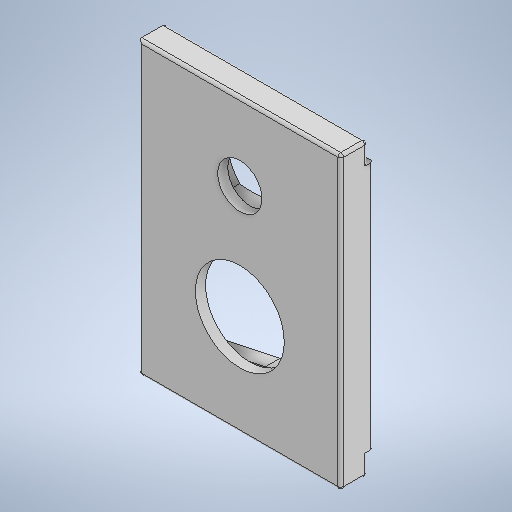
# Autodesk Inventor part: 1mL + 20 mL Luer-Lok 001
Saved by Autodesk Inventor 2025 (Build 290162000, 162)
## iProperties
Created: 2024-04-08
Part Number: 1mL + 20 mL Luer-Lok 001
Material: Generisch
Document SubType Name: Modeling
Designer: noahm
Density: 1 g/cm^3
Appearance: Vorgabe
Author: noahm
Autodesk Inventor part; units mm, degrees
ref_plane "YZ Plane" through (0, 0, 0) normal (1, 0, 0) x (0, 1, 0)
ref_plane "XZ Plane" through (0, 0, 0) normal (0, 1, 0) x (-1, 0, 0)
ref_plane "XY Plane" through (0, 0, 0) normal (0, 0, 1) x (1, 0, 0)
sketch "Skizze1" plane through (0, 0, 0) normal (0, 1, 0) x (-1, 0, 0)
  line L0 (-25, -36) -> (25, -36)
  line L1 (25, -36) -> (25, 36)
  line L2 (25, 36) -> (-25, 36)
  line L3 (-25, 36) -> (-25, -36)
  line L4 (-25, -36) -> (25, 36) construction
  line L5 (25, -36) -> (-25, 36) construction
  circle A0 centre (0, 17) radius 5.5
  circle A1 centre (0, -11) radius 11
  point P0 (0, 0)
  point P1 (0, 36)
  point P2 (0, -36)
  dimension "d0" = 72
  dimension "d1" = 50
  dimension "d2" = 11
  dimension "d3" = 19
  dimension "d4" = 25
  dimension "d5" = 22
  dimension "d6" = 25
  dimension "d7" = 25
  constraints: 12 end point, 4 midpoint, 2 centre point, 2 parallel, 1 horizontal, 1 perpendicular
  measures "d0" distance of L0.end L1.end
  measures "d1" distance of L1.end L2.end
  measures "d2" diameter of A0
  measures "d3" distance of point (0, 36) A0.centre
  measures "d4" distance from line of L1 A0.centre
  measures "d5" diameter of A1
  measures "d6" distance of point (0, -36) A1.centre
  measures "d7" distance from line of L1 A1.centre
extrude "Extrusion1" add sketch "Skizze1" along normal blind 2.5
sketch "Skizze2" plane through (0, 2.5, 0) normal (0, 1, 0) x (1, 0, 0)
  circle A0 centre (0, 11) radius 11
  circle A1 centre (0, -17) radius 5.5
  line L0 (-8.046738, -9.5) -> (0, -10.112591)
  line L1 (0, -10.112591) -> (8.046738, -9.5)
  line L2 (12.459936, -4) -> (0, -3.051436)
  line L3 (0, -3.051436) -> (-12.459936, -4)
  line L4 (-8.046738, -24.5) -> (0, -23.906364)
  line L5 (0, -23.906364) -> (8.046738, -24.5)
  line L6 (-12.459936, 26) -> (0, 25.080787)
  line L7 (0, 25.080787) -> (12.459936, 26)
  arc A2 (8.046738, -24.5) -> (8.046738, -9.5) centre (0, -17) ccw
  arc A3 (-8.046738, -9.5) -> (-8.046738, -24.5) centre (0, -17) ccw
  arc A4 (12.459936, -4) -> (12.459936, 26) centre (0, 11) ccw
  arc A5 (-12.459936, 26) -> (-12.459936, -4) centre (0, 11) ccw
  line L8 (-25, -36) -> (25, -36)
  line L9 (-25, 36) -> (-25, -36)
  line L10 (25, -36) -> (-25, -36)
  line L11 (-25, -36) -> (-25, 36)
  line L12 (-25, 36) -> (25, 36)
  line L13 (25, 36) -> (25, -36)
  point P0 (0, 0)
  point P1 (0, -9.5)
  point P2 (0, -24.5)
  point P3 (0, 26)
  dimension "d12" = 0
  dimension "d13" = 0
  dimension "d14" = 7.5
  dimension "d16" = 7.5
  dimension "d17" = 15
  constraints: 24 end point, 8 point on circle, 6 parallel, 4 centre point, 1 horizontal, 1 perpendicular, 1 vertical alignment
  measures "d12" distance of point (0, 11) A4.centre
  measures "d13" distance of A1.centre A2.centre
  measures "d14" distance of A2.centre point (0, -9.5)
  measures "d16" distance of A2.centre point (0, -24.5)
  measures "d17" distance of A4.centre point (0, 26)
extrude "Extrusion2" add sketch "Skizze2" along normal blind 1.7 contours L9 L12 L13 L8
sketch "Skizze3" plane through (0, 4.2, 0) normal (0, 1, 0) x (1, 0, 0)
  line L0 (-25, -36) -> (25, -36) projected
  line L1 (25, 36) -> (-25, 36) projected
  line L2 (-25, -36) -> (25, -36)
  line L3 (25, -36) -> (25, 36)
  line L4 (25, 36) -> (-25, 36)
  line L5 (-25, 36) -> (-25, -36)
  point P0 (0, 0)
  constraints: 8 end point, 2 parallel, 1 horizontal, 1 perpendicular
extrude "Extrusion3" add sketch "Skizze3" along normal blind 3.8
sketch "Skizze4" plane through (0, 8, 0) normal (0, 1, 0) x (1, 0, 0)
  arc A0 (-8.046738, -9.5) -> (-10.944133, -18.107223) centre (0, -17) ccw
  arc A1 (8.046738, -24.5) -> (10.994414, -16.649483) centre (0, -17) ccw
  arc A2 (0.069499, -10.122825) -> (-0.070045, -10.107258) centre (-0.221864, -12.101488) ccw
  arc A3 (132.908051, -33.706836) -> (133.210878, -29.728206) centre (132.919515, -31.706869) ccw
  arc A4 (12.459811, -3.99999) -> (19.29294, 13.833232) centre (-0.000137, 11) ccw
  line L0 (12.459811, -3.99999) -> (12.459936, -4)
  arc A5 (-4.699403, -1.782332) -> (-4.576398, -1.84238) centre (-3.76103, -0.016134) ccw
  arc A6 (4.726856, 23.857004) -> (4.581609, 23.857004) centre (4.654232, 21.858323) ccw
  arc A7 (0.173536, 25.036036) -> (-0.178728, 25.093972) centre (-0.325875, 23.099393) ccw
  arc A8 (-0.17125, -3.007275) -> (0.176342, -3.064861) centre (0.328161, -1.070632) ccw
  line L1 (19.293045, 13.832979) -> (19.293151, 13.832726) construction
  spline S0 degree 2 poles (19.29294, 13.833232) (19.293045, 13.832979) (19.293151, 13.832726) knots 0 0 0 1 1 1
  line L2 (19.293151, 13.832726) -> (19.293006, 13.832782)
  line L3 (-1.683069, 21.870477) -> (-1.988258, 21.987421)
  arc A9 (12.459936, -4) -> (19.293151, 13.832726) centre (0, 11) ccw
  arc A10 (-12.459936, 26) -> (-19.465197, 9.835475) centre (0, 11) ccw
  line L4 (-2.63509, -24) -> (-2.613775, -24.002826) construction
  spline S1 degree 2 poles (-2.63509, -24) (-2.613775, -24.002826) (-2.592502, -24.005641) knots 0 0 0 1 1 1
  line L5 (2.590414, -10) -> (2.622634, -9.912932)
  line L6 (2.625489, -10.025506) -> (2.590414, -10)
  line L7 (-2.63509, -24) -> (-3.652778, -23.822078) construction
  line L8 (-3.652778, -23.822078) -> (-10.555962, -19.321714) construction
  line L9 (-10.555962, -19.321714) -> (-10.944133, -18.107223) construction
  spline S2 degree 3 poles (-2.63509, -24) (-3.652778, -23.822078) (-10.555962, -19.321714) (-10.944133, -18.107223) knots 1 1 1 1 2 2 2 2
  line L10 (-2.613775, -24.002826) -> (-2.592502, -24.005641) construction
  line L11 (-2.613775, -24.002826) -> (-2.047447, -24.5) construction
  line L12 (-2.047447, -24.5) -> (7.063429, -25.007938) construction
  line L13 (7.063429, -25.007938) -> (8.046738, -24.5) construction
  spline S3 degree 3 poles (-2.613775, -24.002826) (-2.047447, -24.5) (7.063429, -25.007938) (8.046738, -24.5) knots 1 1 1 1 2 2 2 2
  line L14 (-8.046738, -9.5) -> (-7.10437, -8.961841) construction
  line L15 (-7.10437, -8.961841) -> (1.902827, -9.5) construction
  line L16 (1.902827, -9.5) -> (2.590414, -10) construction
  spline S4 degree 3 poles (-8.046738, -9.5) (-7.10437, -8.961841) (1.902827, -9.5) (2.590414, -10) knots 1 1 1 1 2 2 2 2
  line L17 (2.625489, -10.025506) -> (3.48361, -9.847387) construction
  line L18 (3.48361, -9.847387) -> (10.59265, -15.534689) construction
  line L19 (10.59265, -15.534689) -> (10.994414, -16.649483) construction
  spline S5 degree 3 poles (2.625489, -10.025506) (3.48361, -9.847387) (10.59265, -15.534689) (10.994414, -16.649483) knots 1 1 1 1 2 2 2 2
  line L20 (19.29294, 13.833232) -> (19.293045, 13.832979) construction
  line L21 (-12.459936, 26) -> (-9.940805, 26.954912) construction
  line L22 (-9.940805, 26.954912) -> (3.464573, 24.825193) construction
  line L23 (3.464573, 24.825193) -> (4.581609, 23.857004) construction
  spline S6 degree 3 poles (-12.459936, 26) (-9.940805, 26.954912) (3.464573, 24.825193) (4.581609, 23.857004) knots 1 1 1 1 2 2 2 2
  line L24 (4.581609, 23.857004) -> (6.229968, 23.857004) construction
  line L25 (6.229968, 23.857004) -> (18.208958, 16.477012) construction
  line L26 (18.208958, 16.477012) -> (19.293045, 13.832979) construction
  spline S7 degree 3 poles (4.581609, 23.857004) (6.229968, 23.857004) (18.208958, 16.477012) (19.293045, 13.832979) knots 1 1 1 1 2 2 2 2
  line L27 (12.459811, -3.99999) -> (12.463093, -3.997578) construction
  spline S8 degree 3 poles (12.459811, -3.99999) (12.463093, -3.997578) (12.46598, -3.995178) (12.468474, -3.992789) knots 0 0 0 0 1 1 1 1
  line L28 (12.463093, -3.997578) -> (12.46598, -3.995178) construction
  line L29 (12.46598, -3.995178) -> (12.468474, -3.992789) construction
  line L30 (-4.699403, -1.782332) -> (-3.368865, -2.794968) construction
  line L31 (-3.368865, -2.794968) -> (10.298011, -4.836702) construction
  line L32 (10.298011, -4.836702) -> (12.46598, -3.995178) construction
  spline S9 degree 3 poles (-4.699403, -1.782332) (-3.368865, -2.794968) (10.298011, -4.836702) (12.46598, -3.995178) knots 1 1 1 1 2 2 2 2
  line L33 (-4.699403, -1.782332) -> (-6.229968, -1.782332) construction
  line L34 (-6.229968, -1.782332) -> (-18.562842, 6.733725) construction
  line L35 (-18.562842, 6.733725) -> (-19.465197, 9.835475) construction
  spline S10 degree 3 poles (-4.699403, -1.782332) (-6.229968, -1.782332) (-18.562842, 6.733725) (-19.465197, 9.835475) knots 1 1 1 1 2 2 2 2
  line L36 (-25, -36) -> (25, -36)
  line L37 (25, -36) -> (25, 36)
  line L38 (-25, -36) -> (25, -36)
  line L39 (25, -36) -> (25, -31)
  line L40 (25, -31) -> (-25, -31)
  line L41 (-25, -31) -> (-25, -36)
  line L42 (-25, 36) -> (-25, -36)
  line L43 (25, 35.805152) -> (-25, 35.805152)
  line L44 (-25, 35.805152) -> (-25, 30.805152)
  line L45 (-25, 30.805152) -> (25, 30.805152)
  line L46 (25, 30.805152) -> (25, 35.805152)
  point P0 (0, 0)
  point P1 (0, -23.906364)
  point P2 (0, -3.051436)
  point P3 (12.465271, -3.995453)
  point P4 (19.29294, 13.833232)
  dimension "d25" = 0
  dimension "d29" = 5
  dimension "d30" = 5
  constraints: 26 end point, 25 point on circle, 11 centre point, 5 coincident, 5 point on line, 4 parallel, 3 equal radius, 3 horizontal, 2 perpendicular, 1 tangent, 33 other
  measures "d25" vertical distance of point (0, 11) A4.centre
  measures "d29" distance of L44.end L43.end
  measures "d30" distance of L36.start L40.end
extrude "Extrusion4" cut sketch "Skizze4" against normal blind 5.5 contours S4 L6 S5 A1 S3 S1 S2 A0 | S9 S10 A10 S6 S7 A4
sketch "Skizze5" plane through (0, 8, 0) normal (0, 1, 0) x (1, 0, 0)
  line L0 (-25, -36) -> (25, -36) projected
  line L1 (25, -36) -> (25, 36) projected
  line L2 (-25, -36) -> (25, -36)
  line L3 (25, -36) -> (25, -30.8)
  line L4 (25, -30.8) -> (-25, -30.8)
  line L5 (-25, -30.8) -> (-25, -36)
  line L6 (-25, 36) -> (25, 36)
  line L7 (25, 36) -> (25, 30.8)
  line L8 (25, 30.8) -> (-25, 30.8)
  line L9 (-25, 30.8) -> (-25, 36)
  line L10 (25, 36) -> (-25, 36) projected
  point P0 (0, 0)
  point P1 (25, 36)
  dimension "d34" = 5.2
  dimension "d35" = 5.2
  dimension "d36" = 5.2
  constraints: 16 end point, 4 parallel, 3 point on line, 2 horizontal, 2 perpendicular
  measures "d34" distance of L0.start L4.end
  measures "d35" distance from line of L10 L8.end
  measures "d36" distance of L8.end L6.start
extrude "Extrusion5" cut sketch "Skizze5" against normal blind 1.375
fillet "Rundung1" radius 0.7 15 edges at (25, 8, 0) (25, 0, 0) (-25, 8, 0) (-25, 0, 0) (0, 6.625, -36) (0, 0, -36) (25, 3.3125, -36) (-25, 3.3125, -36) (25, 3.3125, 36) (25, 6.625, 33.4) (-25, 6.625, 33.4) (0, 6.625, 36) (0, 0, 36) (25, 6.625, -33.4) (-25, 6.625, -33.4)
sketch "Skizze6" plane through (0, 8, 0) normal (0, 1, 0) x (1, 0, 0)
  circle A0 centre (0, 11) radius 12.1
  circle A1 centre (0, 11) radius 11
  arc A2 (-12.459936, 26) -> (-19.465197, 9.835475) centre (0, 11) ccw
  line L0 (-19.465197, 9.835475) -> (-6.928142, 1.079776)
  line L1 (12.459936, -4) -> (-2.890427, -0.749699)
  line L2 (-12.459936, 26) -> (3.045711, 22.710407)
  arc A3 (12.459936, -4) -> (12.459936, 26) centre (0, 11) ccw
  arc A4 (-19.465197, 9.835475) -> (12.459936, -4) centre (0.596699, 12.376874) ccw
  line L3 (19.292862, 13.83469) -> (6.049078, 21.479439)
  arc A5 (19.292862, 13.83469) -> (-12.459936, 26) centre (0, 11) ccw
  point P0 (0, 0)
  point P1 (1.971471, 22.938312)
  point P2 (-2.119904, -0.912851)
  dimension "d40" = 24.2
  dimension "d41" = 0
  constraints: 9 point on circle, 8 end point, 3 centre point, 2 tangent, 1 concentric, 1 vertical alignment
  measures "d40" diameter of A0
  measures "d41" distance of point (0, 11) A0.centre
extrude "Extrusion6" add sketch "Skizze6" against normal blind 3.7 contours A0 L1 L2 | A0 L2 A5 A3 L3 | L1 A4 L0 A0 | A0 L1 | L2 A0 | A1
sketch "Skizze7" plane through (0, 8, 0) normal (0, 1, 0) x (1, 0, 0)
  circle A0 centre (0, 11) radius 12.1
  arc A1 (1.971471, 22.938312) -> (-6.928142, 1.079776) centre (0, 11) ccw
  point P0 (0, 0)
  dimension "d44" = 24.2
  dimension "d45" = 0
  constraints: 1 centre point
  measures "d44" diameter of A0
  measures "d45" distance of A1.centre A0.centre
extrude "Extrusion7" cut sketch "Skizze7" against normal blind 3.7
